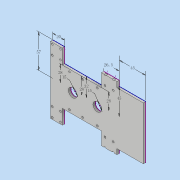
# Autodesk Inventor part: 底盘4.0
Saved by Autodesk Inventor 2019 (Build 230136000, 136)
## iProperties
Created: 2020-11-02
Part Number: 底盘4.0
Material: Generic
Document SubType Name: Modeling
Designer: Wang Hua
Density: 1 g/cm^3
Appearance: Default
Author: Wang Hua
Autodesk Inventor part; units mm, degrees
ref_plane "YZ Plane" through (0, 0, 0) normal (1, 0, 0) x (0, 1, 0)
ref_plane "XZ Plane" through (0, 0, 0) normal (0, 1, 0) x (-1, 0, 0)
ref_plane "XY Plane" through (0, 0, 0) normal (0, 0, 1) x (1, 0, 0)
sketch "草图1" plane through (0, 0, 0) normal (0, 0, 1) x (1, 0, 0)
  line L0 (-144.4444, 0) -> (-144.4444, 57)
  line L1 (-144.4444, 57) -> (-124.4444, 57)
  line L2 (-124.4444, 57) -> (-124.4444, 32)
  line L3 (-124.4444, 32) -> (-57.6944, 32)
  line L4 (-57.6944, 32) -> (-57.6944, 54)
  line L5 (-57.6944, 54) -> (-31.1944, 54)
  line L6 (-31.1944, 54) -> (-31.1944, 45)
  line L7 (-31.1944, 45) -> (13.8056, 45)
  line L8 (13.8056, 45) -> (13.8056, 0)
  line L9 (0, 0) -> (-166.6667, 0) construction
  line L10 (-144.4444, 0) -> (-144.4444, -57)
  line L11 (-144.4444, -57) -> (-124.4444, -57)
  line L12 (-124.4444, -57) -> (-124.4444, -32)
  line L13 (-124.4444, -32) -> (-57.6944, -32)
  line L14 (-57.6944, -32) -> (-57.6944, -54)
  line L15 (-57.6944, -54) -> (-31.1944, -54)
  line L16 (-31.1944, -54) -> (-31.1944, -45)
  line L17 (-31.1944, -45) -> (13.8056, -45)
  line L18 (13.8056, -45) -> (13.8056, 0)
  circle A0 centre (-106.5528, 0) radius 7.5
  circle A1 centre (-64.5976, 0) radius 7.5
  point P0 (-141.4444, -54)
  point P1 (-127.4444, -54)
  point P2 (-51.4444, -54)
  point P3 (-37.4444, -54)
  point P4 (-112.1204, -28)
  point P5 (-64.5976, -28)
  point P6 (-89.6514, -28)
  point P7 (-127.4444, -38)
  point P8 (-141.4444, -38)
  point P9 (-51.4444, -38)
  point P10 (-37.4444, -38)
  point P11 (-141.4444, 54)
  point P12 (-127.4444, 54)
  point P13 (-127.4444, 38)
  point P14 (-141.4444, 38)
  point P15 (-51.4444, 54)
  point P16 (-51.4444, 38)
  point P17 (-37.4444, 54)
  point P18 (-37.4444, 38)
  point P19 (-64.5976, 28)
  point P20 (-89.6514, 28)
  point P21 (-112.1204, 28)
  dimension "d0" = 20
  dimension "d1" = 26.5
  dimension "d3" = 32
  dimension "d4" = 45
  dimension "d5" = 45
  dimension "d6" = 57
  dimension "d7" = 15
  dimension "d8" = 15
  dimension "d29" = 28
  dimension "d30" = 28
  dimension "d31" = 28
  constraints: 38 end point, 19 symmetric about line, 7 perpendicular, 4 point on line, 2 centre point, 2 vertical, 1 horizontal
  measures "d0" distance of L0.end L1.end
  measures "d1" distance of L4.end L5.end
  measures "d3" distance between parallel lines of L9 L3
  measures "d4" distance between parallel lines of L9 L7
  measures "d5" distance of L6.end L7.end
  measures "d6" distance of L0.start L0.end
  measures "d7" diameter of A0
  measures "d8" diameter of A1
  measures "d29" distance from line of L9 point (-112.12, 28)
  measures "d30" distance from line of L9 point (-89.651, 28)
  measures "d31" distance from line of L9 point (-64.598, 28)
extrude "拉伸1" add sketch "草图1" along normal blind 4
hole "孔1" at (-141.4444, -54, 0) at (-127.4444, -54, 0) at (-127.4444, -38, 0) at (-141.4444, -38, 0) at (-51.4444, -54, 0) at (-51.4444, -38, 0) at (-37.4444, -54, 0) at (-37.4444, -38, 0) at (-64.5976, -28, 0) at (-89.6514, -28, 0) at (-112.1204, -28, 0) at (-141.4444, 38, 0) at (-127.4444, 54, 0) at (-141.4444, 54, 0) at (-127.4444, 38, 0) at (-112.1204, 28, 0) at (-89.6514, 28, 0) at (-64.5976, 28, 0) at (-51.4444, 38, 0) at (-37.4444, 38, 0) at (-37.4444, 54, 0) at (-51.4444, 54, 0) direction (0, 0, 1) diameter 3.2 end through all
